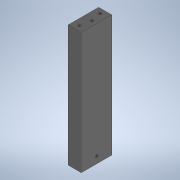
# Autodesk Inventor part: shin2x4
Saved by Autodesk Inventor 2021.5 (Build 255421000, 421)
## iProperties
Created: 2024-11-18
Part Number: shin2x4
Material: Wood (Birch)
Document SubType Name: Modeling
Designer: email
Density: 0.55 g/cm^3
Appearance: Birch - Natural Polished
Author: email
Autodesk Inventor part; units mm, degrees
ref_plane "YZ Plane" through (0, 0, 0) normal (1, 0, 0) x (0, 1, 0)
ref_plane "XZ Plane" through (0, 0, 0) normal (0, 1, 0) x (-1, 0, 0)
ref_plane "XY Plane" through (0, 0, 0) normal (0, 0, 1) x (1, 0, 0)
sketch "Sketch1" plane through (0, 0, 0) normal (0, 1, 0) x (-1, 0, 0)
  line L0 (0, 0) -> (-38.1, 0)
  line L1 (-38.1, 0) -> (-38.1, -88.9)
  line L2 (-38.1, -88.9) -> (0, -88.9)
  line L3 (0, -88.9) -> (0, 0)
  dimension "d0" = 38.1
  dimension "d1" = 88.9
  constraints: 8 end point, 2 parallel, 1 horizontal, 1 perpendicular
  measures "d0" distance of L1.end L2.end
  measures "d1" distance of L0.end L1.end
extrude "Extrusion1" add sketch "Sketch1" along normal blind 355.6
sketch "Sketch3" plane through (0, 355.6, 0) normal (0, 1, 0) x (1, 0, 0)
  line L0 (0, 88.9) -> (0, 0) projected
  line L1 (0, 74.725) -> (18.45, 74.725)
  line L2 (18.45, 74.725) -> (18.45, 0) construction
  line L3 (18.45, 0) -> (0, 0)
  line L4 (0, 0) -> (0, 74.725)
  line L5 (38.1, 88.9) -> (0, 88.9) projected
  line L6 (18.45, 74.725) -> (18.45, 61.2)
  line L7 (18.45, 74.725) -> (18.45, 14.175)
  line L8 (18.45, 44.45) -> (24.45, 44.45)
  line L9 (0, 0) -> (38.1, 0) projected
  dimension "d35" = 60.55
  dimension "d42" = 6
  dimension "d43" = 30.275
  dimension "d45" = 14.175
  dimension "d46" = 14.175
  dimension "d48" = 24.45
  dimension "d49" = 44.45
  constraints: 14 end point, 3 point on line, 2 parallel, 2 perpendicular, 1 horizontal, 1 midpoint
  measures "d35" distance of L7.end L1.end
  measures "d42" distance of L8.start L8.end
  measures "d43" distance from line of L1.end L8
  measures "d45" distance from line of L5 L1.end
  measures "d46" distance from line of L9 L7.end
  measures "d48" distance from line of L0 L8.end
  measures "d49" distance between parallel lines of L5 L8
hole "Hole1" at (18.45, 355.6, -74.725) at (24.45, 355.6, -44.45) at (18.45, 355.6, -14.175) direction (0, -1, 0) diameter 7 depth 10 tip angle 118
sketch "Sketch4" plane through (38.1, 0, 0) normal (1, 0, 0) x (0, 0, -1)
  line L0 (0, 0) -> (88.9, 0) projected
  line L1 (0, 0) -> (44.45, 0) construction
  line L2 (44.45, 0) -> (44.45, 20) construction
  line L3 (44.45, 20) -> (0, 20) construction
  line L4 (0, 20) -> (0, 0) construction
  dimension "d25" = 44.45
  dimension "d26" = 20
  constraints: 8 end point, 2 parallel, 1 horizontal, 1 perpendicular
  measures "d25" distance between parallel lines of L4 L2
  measures "d26" distance between parallel lines of L0 L3
hole "Hole2" at (38.1, 20, -44.45) direction (-1, 0, 0) diameter 6.5 depth 10
body "Solid1"
